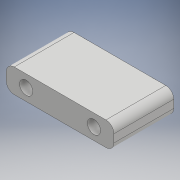
# Autodesk Inventor part: FixLock
Saved by Autodesk Inventor 2017 (Build 210142000, 142)
## iProperties
Created: 2017-07-10
Part Number: FixLock
Material: Generic
Document SubType Name: Modeling
Designer: beat
Density: 1 g/cm^3
Appearance: Default
Author: beat
Autodesk Inventor part; units mm, degrees
ref_plane "YZ Plane" through (0, 0, 0) normal (1, 0, 0) x (0, 1, 0)
ref_plane "XZ Plane" through (0, 0, 0) normal (0, 1, 0) x (-1, 0, 0)
ref_plane "XY Plane" through (0, 0, 0) normal (0, 0, 1) x (1, 0, 0)
sketch "Sketch1" plane through (0, 0, 0) normal (0, 1, 0) x (-1, 0, 0)
  line L0 (-13.5, 3) -> (13.5, 3)
  line L1 (13.5, 3) -> (13.5, -3)
  line L2 (13.5, -3) -> (-13.5, -3)
  line L3 (-13.5, -3) -> (-13.5, 3)
  line L4 (-13.5, 3) -> (13.5, -3) construction
  line L5 (13.5, 3) -> (-13.5, -3) construction
  point P0 (0, 0)
  dimension "d0" = 27
  dimension "d1" = 6
  constraints: 12 end point, 2 midpoint, 2 parallel, 1 horizontal, 1 perpendicular
  measures "d0" distance of L1.end L2.end
  measures "d1" distance of L0.end L1.end
extrude "Extrusion1" add sketch "Sketch1" along normal blind 15
sketch "Sketch2" plane through (0, 15, 0) normal (0, 1, 0) x (1, 0, 0)
  line L0 (-8.5, 0) -> (8.5, 0)
  point P0 (0, 0)
  point P1 (0, 0)
  dimension "d4" = 17
  constraints: 2 end point, 1 coincident, 1 horizontal, 1 midpoint
  measures "d4" distance of L0.start L0.end
hole "Hole1" at (-8.5, 15, 0) at (8.5, 15, 0) direction (0, -1, 0) diameter 3.3 end through all countersink diameter 6 countersink angle 90
fillet "Fillet1" radius 2 4 edges at (-13.5, 7.5, 3) (-13.5, 7.5, -3) (13.5, 7.5, -3) (13.5, 7.5, 3)
body "Solid1"
